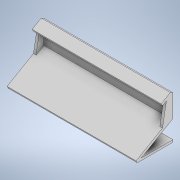
# Autodesk Inventor part: Name_card_case
Saved by Autodesk Inventor 2020 (Build 240168000, 168)
## iProperties
Created: 2020-09-20
Part Number: Name_card_case
Material: Generic
Document SubType Name: Modeling
Designer: maple
Density: 1 g/cm^3
Appearance: Default
Author: maple
Autodesk Inventor part; units mm, degrees
ref_plane "YZ Plane" through (0, 0, 0) normal (1, 0, 0) x (0, 1, 0)
ref_plane "XZ Plane" through (0, 0, 0) normal (0, 1, 0) x (-1, 0, 0)
ref_plane "XY Plane" through (0, 0, 0) normal (0, 0, 1) x (1, 0, 0)
sketch "Sketch1" plane through (0, 0, 0) normal (1, 0, 0) x (0, 1, 0)
  line L0 (0, 0) -> (17, 0)
  line L1 (17, 0) -> (17, -2)
  line L2 (17, -2) -> (0, -2)
  line L3 (0, -2) -> (0, 0)
  line L4 (17, 0) -> (13, 6.9282)
  line L5 (17, 0) -> (25, 0) construction
  line L6 (13, 6.9282) -> (11.2679, 5.9282)
  line L7 (11.2679, 5.9282) -> (14.6906, 0)
  line L8 (0, 0) -> (-15, 25.9808)
  line L9 (0, 0) -> (30, 0) construction
  line L10 (-15, 25.9808) -> (-16.7321, 24.9808)
  line L11 (-16.7321, 24.9808) -> (-1.1547, -2)
  line L12 (-1.1547, -2) -> (0, -2)
  line L13 (-16.7321, 24.9808) -> (-16.7321, -2)
  line L14 (-15, 25.9808) -> (-15, -2)
  line L15 (-15, -2) -> (-16.7321, -2)
  line L16 (17, 0) -> (15.8453, -2)
  point P0 (-15, 21.9808)
  dimension "d0" = 17
  dimension "d1" = 2
  dimension "d2" = 8
  dimension "d3" = 120
  dimension "d4" = 2
  dimension "d5" = 30
  dimension "d6" = 120
  dimension "d7" = 2
  constraints: 34 end point, 7 perpendicular, 4 horizontal, 3 parallel, 3 point on line, 2 equal length, 1 vertical
  measures "d0" distance of L1.end L2.end
  measures "d1" distance of L0.end L1.end
  measures "d2" distance of L0.end L4.end
  measures "d3" angle of L5 L4
  measures "d4" distance of L4.end L6.end
  measures "d5" distance of L0.start L8.end
  measures "d6" angle of L9 L8
  measures "d7" distance of L8.end L10.end
extrude "Extrusion1" add sketch "Sketch1" along normal blind 98 contours L0 L16 L2 L3 | L3 L12 L11 L14 L8 | L7 L6 L4 L0 | L14 L11 L10 | L11 L14 L15 L13
sketch "Sketch2" plane through (98, 0, 0) normal (1, 0, 0) x (0, 0, -1)
  line L0 (-5.9282, 11.2679) -> (-5.9282, -3.4226)
  line L1 (0, 0) -> (-25.9808, -15) projected
  line L2 (-5.9282, -3.4226) -> (-2.9641, 12.9793)
  line L3 (-5.9282, 11.2679) -> (0, 14.6906) projected
  line L4 (-5.9282, -3.4226) -> (0, 0)
  line L5 (0, 0) -> (0, 14.6906)
  line L6 (-2.9641, 12.9793) -> (0, 14.6906)
  constraints: 10 end point, 2 vertical, 1 collinear, 1 midpoint, 1 point on line
extrude "Extrusion2" add sketch "Sketch2" against normal blind 2 contours L2 L3 L5 L1
sketch "Sketch3" plane through (0, 0, 0) normal (-1, 0, 0) x (0, 0, 1)
  line L0 (2.9641, 12.9793) -> (5.9282, -3.4226) projected
  line L1 (5.9282, -3.4226) -> (2.9641, 12.9793)
  line L2 (5.9282, 11.2679) -> (0, 14.6906) projected
  line L3 (2.9641, 12.9793) -> (0, 14.6906)
  line L4 (5.9282, -3.4226) -> (0, 0) projected
  line L5 (0, 14.6906) -> (0, 0)
  line L6 (0, 0) -> (5.9282, -3.4226)
  constraints: 8 end point, 3 collinear, 1 vertical
extrude "Extrusion3" add sketch "Sketch3" against normal blind 2
body "Solid1"
